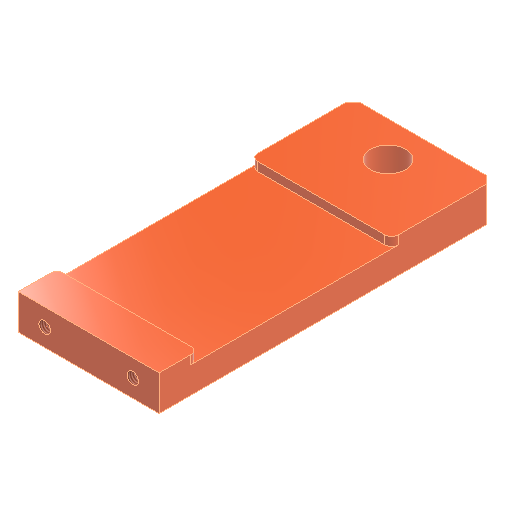
# Autodesk Inventor part: GRJ-03-114
Saved by Autodesk Inventor 2026.1 (Build 301233000, 233)
## iProperties
Company: Gree
Created: 2024-12-19
Part Number: GRJ-03-114
Material: Fenolite OR
Document SubType Name: Modeling
Designer: Willian Pinheiro
Density: 1.38 g/cm^3
Appearance: Suave - Laranja claro
Description: Coluna Eixo
Mass: 43.5581 g
Surface Area: 107.132 cm^2
Volume: 31.5638 cm^3
Project: GRJ-03
Checked By: Antonio Lucas
Engr Approved By: Antonio Lucas
Mfg Approved By: Anderson Oliveira
Dimensões: 10 x 40 x 95 mm
Total: 2
Author: Willian Pinheiro
Revision Number: 00
Title: Soldagem
Autodesk Inventor part; units mm, degrees
ref_plane "YZ Plane" through (0, 0, 0) normal (1, 0, 0) x (0, 1, 0)
ref_plane "XZ Plane" through (0, 0, 0) normal (0, 1, 0) x (-1, 0, 0)
ref_plane "XY Plane" through (0, 0, 0) normal (0, 0, 1) x (1, 0, 0)
sketch "Esboço1" plane through (0, 0, 0) normal (0, 0, 1) x (1, 0, 0)
  line L0 (-20, -47.5) -> (20, -47.5)
  line L1 (20, -47.5) -> (20, 47.5)
  line L2 (20, 47.5) -> (-20, 47.5)
  line L3 (-20, 47.5) -> (-20, -47.5)
  line L4 (-20, 47.5) -> (20, 47.5)
  circle A0 centre (0, 37.5) radius 5
  circle A1 centre (0, 37.5) radius 27.5862 construction
  circle A2 centre (0, 37.5) radius 74 construction
  line L5 (-20, 18.5) -> (20, 18.5)
  line L6 (-20, -36.5) -> (20, -36.5)
  line L7 (-103.6, 0) -> (103.6, 0) construction
  line L8 (0, -79.3) -> (0, 143.3) construction
  point P0 (0, 0)
  dimension "d0" = 95
  dimension "d1" = 40
  dimension "d41" = 10
  dimension "d42" = 85
  dimension "d43" = 55.1725
  dimension "d45" = 84
  dimension "d49" = 66
  constraints: 14 end point, 5 point on line, 3 centre point, 3 parallel, 2 coincident, 2 horizontal, 2 point on circle, 1 perpendicular, 1 tangent, 2 other
  measures "d0" distance between parallel lines of L0 L2
  measures "d1" distance of L2.end L1.end
  measures "d41" diameter of A0
  measures "d42" distance from line of L0 A0.centre
  measures "d43" diameter of A1
  measures "d49" distance between parallel lines of L0 L5
extrude "Extrusão1" add sketch "Esboço1" along normal mid plane 10 contours L3 L6 L1 L0 | L3 L5 L1 L6 | L3 L2 L1 L5 | A0
extrude "Extrusão4" cut sketch "Esboço1" against normal blind 2.5 from surface at 5 contours L3 L5 L1 L6
sketch "Esboço2" plane through (-20, -47.5, -5) normal (0, -1, 0) x (1, 0, 0)
  line L0 (40, 10) -> (40, 0)
  line L1 (40, 5) -> (0, 5) construction
  line L2 (0, 0) -> (0, 10)
  line L3 (0, 0) -> (0, 10) projected
  line L4 (40, 0) -> (40, 10) projected
  line L5 (0, 10) -> (40, 10) construction
  line L6 (20, 10) -> (20, 0) construction
  line L7 (40, 0) -> (0, 0) construction
  point P0 (20, 5)
  point P1 (7.5, 5)
  point P2 (32.5, 5)
  dimension "d9" = 7.5
  dimension "d10" = 7.5
  dimension "d37" = 25
  constraints: 8 end point, 4 midpoint, 2 point on line, 1 symmetric about line
  measures "d9" distance from line of L2 point (7.5, 5)
  measures "d10" distance from line of L0 point (32.5, 5)
  measures "d37" distance of point (32.5, 5) point (7.5, 5)
hole "Furo1" at (-12.5, -47.5, 0) at (12.5, -47.5, 0) direction (0, 1, 0) diameter 3.242 depth 15 tip angle 118 thread size "M4x0.7" class "6H" standard "ISO Metric profile"
sketch "Esboço3" plane through (0, 0, 5) normal (0, 0, 1) x (1, 0, 0)
  point P0 (0, 0)
  point P1 (0, 37.5)
  point P2 (0, 37.5)
hole "Furo2" at (0, 37.5, 5) direction (0, 0, -1) diameter 6 end through all counterbore diameter 10 counterbore depth 7
fillet "Arredondamento3" radius 2 4 edges at (-20, 18.5, 3.75) (20, 18.5, 3.75) (-20, -36.5, 3.75) (20, -36.5, 3.75)
chamfer "Chanfro2" distance 2 angle 45 2 edges at (-20, 47.5, 0) (20, 47.5, 0)
